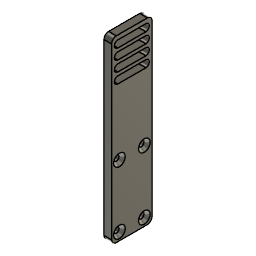
laser_mount (Autodesk Fusion 360 design; units mm, degrees)
Autodesk Fusion 360 part; units mm, degrees
sketch "Sketch1" plane through (0, 0, 0) normal (1, 0, 0) x (0, 1, 0)
  line L0 (-13, 57.5) -> (13, 57.5)
  line L1 (13, 57.5) -> (13, -57.5)
  line L2 (13, -57.5) -> (-13, -57.5)
  line L3 (-13, -57.5) -> (-13, 57.5)
  line L4 (-13, 57.5) -> (13, -57.5) construction
  line L5 (13, 57.5) -> (-13, -57.5) construction
  circle A0 centre (-8, -12.5) radius 1.75
  circle A1 centre (8, -12.5) radius 1.75
  circle A2 centre (8, -52.5) radius 1.75
  circle A3 centre (-8, -52.5) radius 1.75
  line L6 (-9, 30.25) -> (9, 30.25)
  arc A4 (9, 30.25) -> (9, 34.75) centre (9, 32.5) ccw
  line L7 (9, 34.75) -> (-9, 34.75)
  arc A5 (-9, 34.75) -> (-9, 30.25) centre (-9, 32.5) ccw
  line L8 (-9, 32.5) -> (9, 32.5) construction
  line L9 (0, 0) -> (0, 10)
  arc A6 (-9, 41.4167) -> (-9, 36.9167) centre (-9, 39.1667) ccw
  line L10 (9, 41.4167) -> (-9, 41.4167)
  line L11 (-9, 39.1667) -> (9, 39.1667) construction
  line L12 (-9, 36.9167) -> (9, 36.9167)
  arc A7 (9, 36.9167) -> (9, 41.4167) centre (9, 39.1667) ccw
  arc A8 (-9, 48.0833) -> (-9, 43.5833) centre (-9, 45.8333) ccw
  line L13 (9, 48.0833) -> (-9, 48.0833)
  line L14 (-9, 45.8333) -> (9, 45.8333) construction
  line L15 (-9, 43.5833) -> (9, 43.5833)
  arc A9 (9, 43.5833) -> (9, 48.0833) centre (9, 45.8333) ccw
  arc A10 (-9, 54.75) -> (-9, 50.25) centre (-9, 52.5) ccw
  line L16 (9, 54.75) -> (-9, 54.75)
  line L17 (-9, 52.5) -> (9, 52.5) construction
  line L18 (-9, 50.25) -> (9, 50.25)
  arc A11 (9, 50.25) -> (9, 54.75) centre (9, 52.5) ccw
  dimension "d1" = 16
  dimension "d2" = 40
  dimension "d3" = 3.5
  dimension "d4" = 5
  dimension "d5" = 8
  dimension "d6" = 5
  dimension "d7" = 70
  dimension "d9" = 4.5
  dimension "d10" = 45
  dimension "d11" = 9
  dimension "d12" = 18
  dimension "d15" = 20
  dimension "d16" = 0
  constraint horizontal L0
  constraint perpendicular L0 L1
  constraint parallel L0 L2
  constraint parallel L1 L3
  constraint coincident L4 L9.start
  constraint coincident L5 L9.start
  constraint coincident L9.start origin
  constraint vertical A0.centre A3.centre
  constraint horizontal A0.centre A1.centre
  constraint horizontal A2.centre A3.centre
  constraint vertical A1.centre A2.centre
  constraint equal A0 A1
  constraint equal A0 A3
  constraint equal A0 A2
  constraint tangent L6 A4
  constraint tangent A4 L7
  constraint parallel L6 L7
  constraint tangent L7 A5
  constraint tangent L6 A5
  constraint horizontal L8
  constraint vertical L9
  measures "d1" distance of A2.centre A3.centre
  measures "d2" distance of A0.centre A3.centre
  measures "d3" diameter of A0
  measures "d4" distance of L2 A3.centre
  measures "d5" horizontal distance of L9.start A2.centre
  measures "d6" distance of L1 A2.centre
  measures "d7" distance of L0 A0.centre
  measures "d9" diameter of A4
  measures "d10" vertical distance of A0.centre A5.centre
  measures "d11" horizontal distance of L9.start A5.centre
  measures "d12" distance of A5.centre A4.centre
extrude "Extrude1" add sketch "Sketch1" along normal blind 5
fillet "Fillet1" radius 3 4 edges at (2.5, -13, 57.5) (2.5, 13, 57.5) (2.5, -13, -57.5) (2.5, 13, -57.5)
chamfer "Chamfer1" distance 2 angle 45 1 edges at (5, -9.6316, -11.8672)
chamfer "Chamfer1" distance 2 angle 45 3 edges at (5, 6.3684, -11.8672) (5, -9.6316, -51.8672) (5, 6.3684, -51.8672)
equation "d5 = ( 16 / 2 ) * 1 mm"
